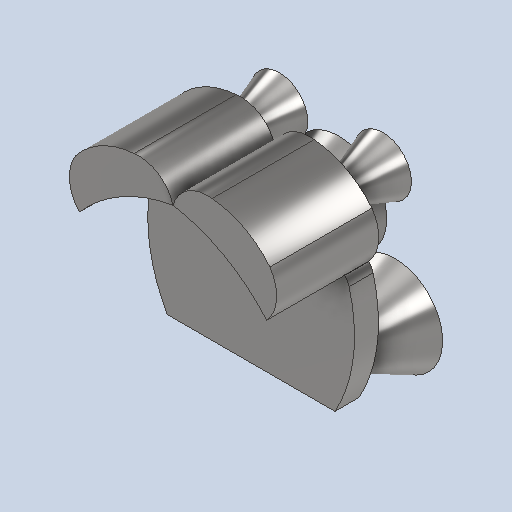
# Autodesk Inventor part: engines
Saved by Autodesk Inventor 2024 (Build 280153000, 153)
## iProperties
Created: 2023-06-07
Part Number: engines
Material: Steel, Mild
Document SubType Name: Modeling
Designer: tamiz
Density: 7.85 g/cm^3
Appearance: Semi-Polished
Author: tamiz
Autodesk Inventor part; units mm, degrees
note: some values were not read from the file. Chosen so that the rebuilt part matches the saved one: second side of "Extrusion11".
ref_plane "YZ Plane" through (0, 0, 0) normal (1, 0, 0) x (0, 1, 0)
ref_plane "XZ Plane" through (0, 0, 0) normal (0, 1, 0) x (-1, 0, 0)
ref_plane "XY Plane" through (0, 0, 0) normal (0, 0, 1) x (1, 0, 0)
sketch "Sketch3" plane through (0, 0, 0) normal (0, 0, 1) x (1, 0, 0)
  line L0 (3200.4, -3619.5) -> (-3200.4, -3619.5)
  line L1 (0, -3619.5) -> (0, 3086.1) construction
  arc A0 (-3738.1541, 769.8538) -> (-3200.4, -3619.5) centre (1884.0877, -768.9648) ccw
  arc A1 (0, 3086.1) -> (-3578.7308, 1068.0837) centre (1038.9488, -2938.6136) ccw
  arc A2 (-3578.7308, 1068.0837) -> (-3738.1541, 769.8538) centre (-3003.1863, 568.6916) ccw
  arc A3 (3200.4, -3619.5) -> (3738.1541, 769.8538) centre (-1884.0877, -768.9648) ccw
  arc A4 (3578.7308, 1068.0837) -> (0, 3086.1) centre (-1038.9488, -2938.6136) ccw
  arc A5 (3738.1541, 769.8538) -> (3578.7308, 1068.0837) centre (3003.1863, 568.6916) ccw
  arc A6 (-3278.4432, 715.8952) -> (-2925.1203, -3162.3) centre (1884.0877, -768.9648) ccw
  line L2 (-2925.1203, -3162.3) -> (2925.1203, -3162.3)
  arc A7 (2925.1203, -3162.3) -> (3278.4432, 715.8952) centre (-1884.0877, -768.9648) ccw
  arc A8 (3278.4432, 715.8952) -> (0, 2621.5927) centre (-1038.9488, -2938.6136) ccw
  arc A9 (0, 2621.5927) -> (-3278.4432, 715.8952) centre (1038.9488, -2938.6136) ccw
  dimension "d3" = 6400.8
  dimension "d4" = 6705.6
  dimension "d5" = 762
  dimension "d6" = 457.2
  constraints: 20 point on circle, 10 centre point, 6 end point, 5 symmetric about line, 2 tangent, 1 midpoint, 1 vertical, 7 other
  measures "d3" distance of L0.start L0.end
  measures "d4" distance of L1.start L1.end
  measures "d5" radius of A2
  measures "d6" radial gap between concentric circles of A1 A9
extrude "Extrusion9" add sketch "Sketch3" against normal blind 914.4 contours L0 A0 A2 A1 A4 A5 A3 | A9 A8 A7 L2 A6
sketch "Sketch14" plane through (0, 0, -914.4) normal (0, 0, -1) x (-1, 0, 0)
  line L0 (0, 3086.1) -> (0, -4176.5904) construction
  arc A0 (-3696.6852, 2888.9142) -> (-3575.8252, 1071.43) centre (-2485.7718, 2056.6775) ccw
  arc A1 (0, 3086.1) -> (-1489.0459, 4049.3399) centre (-1299.2098, 2710.2449) ccw
  arc A2 (-1489.0459, 4049.3399) -> (-3696.6852, 2888.9142) centre (-1247.1211, 908.9303) ccw
  arc A3 (3575.8252, 1071.43) -> (3696.6852, 2888.9142) centre (2485.7718, 2056.6775) ccw
  arc A4 (1489.0459, 4049.3399) -> (0, 3086.1) centre (1299.2098, 2710.2449) ccw
  arc A5 (3696.6852, 2888.9142) -> (1489.0459, 4049.3399) centre (1247.1211, 908.9303) ccw
  arc A6 (3578.7308, 1068.0837) -> (0, 3086.1) centre (-1038.9488, -2938.6136) ccw projected
  arc A7 (3578.7308, 1068.0837) -> (0, 3086.1) centre (-1038.9488, -2938.6136) ccw
  arc A8 (0, 3086.1) -> (-3578.7308, 1068.0837) centre (1038.9488, -2938.6136) ccw projected
  arc A9 (-3578.7308, 1068.0837) -> (-3738.1541, 769.8538) centre (-3003.1863, 568.6916) ccw projected
  arc A10 (0, 3086.1) -> (-3578.7308, 1068.0837) centre (1038.9488, -2938.6136) ccw
  constraints: 17 point on circle, 8 centre point, 6 symmetric about line, 2 end point, 1 point on line, 1 vertical, 3 other
extrude "Extrusion11" add sketch "Sketch14" against normal blind 3895.344
sketch "Sketch15" plane through (0, 0, -914.4) normal (0, 0, -1) x (-1, 0, 0)
  circle A0 centre (-1978.2373, 2378.6391) radius 305.71
  circle A1 centre (-1978.2373, 2378.6391) radius 182.88
  point P0 (0, 0)
  dimension "d61" = 611.42
  dimension "d63" = 365.76
  constraints: 2 centre point, 1 coincident
  measures "d61" diameter of A0
  measures "d63" diameter of A1
extrude "Extrusion12" add sketch "Sketch15" along normal blind 2139.696 draft 20 contours A0 | A1
extrude "Extrusion13" cut sketch "Sketch15" along normal blind 2139.696 draft 20 contours A1
mirror "Mirror2" about plane through (0, 0, 0) normal (1, 0, 0) of "Extrusion12", "Extrusion13"
sketch "Sketch17" plane through (0, 0, -914.4) normal (0, 0, -1) x (-1, 0, 0)
  circle A0 centre (0, 381.214) radius 685.8
  circle A1 centre (-2133.6, -2593.7489) radius 685.8
  circle A2 centre (2133.6, -2593.7489) radius 685.8
  circle A3 centre (0, 381.214) radius 533.4
  circle A4 centre (2133.6, -2593.7489) radius 533.4
  circle A5 centre (-2133.6, -2593.7489) radius 533.4
  point P0 (0, 0)
  dimension "d74" = 1371.6
  dimension "d75" = 1371.6
  dimension "d76" = 1371.6
  dimension "d79" = 1066.8
  dimension "d80" = 1066.8
  dimension "d81" = 1066.8
  constraints: 6 centre point, 3 coincident
  measures "d74" diameter of A0
  measures "d75" diameter of A1
  measures "d76" diameter of A2
  measures "d79" diameter of A3
  measures "d80" diameter of A4
  measures "d81" diameter of A5
extrude "Extrusion14" add sketch "Sketch17" along normal blind 2438.4 draft 25 contours A0 | A1 | A2 | A3 | A4 | A5
extrude "Extrusion15" cut sketch "Sketch17" along normal blind 2438.4 draft 25 contours A3 | A4 | A5
body "Solid2"
